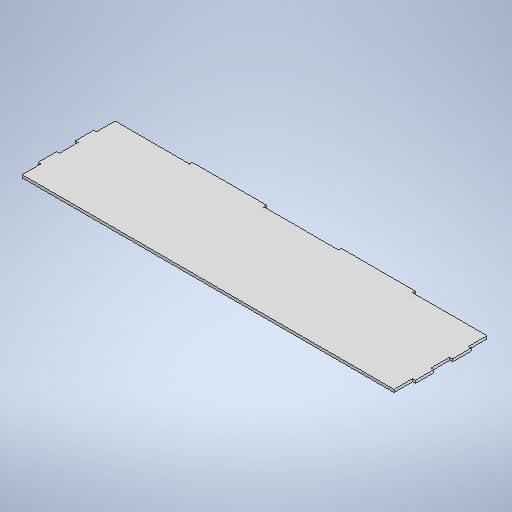
# Autodesk Inventor part: Estante int
Saved by Autodesk Inventor 2025.1 (Build 291241020, 241B)
## iProperties
Created: 2024-11-13
Part Number: Estante int
Material: Generic
Document SubType Name: Modeling
Designer: marco
Density: 1 g/cm^3
Appearance: Default
Author: marco
Autodesk Inventor part; units mm, degrees
ref_plane "YZ Plane" through (0, 0, 0) normal (1, 0, 0) x (0, 1, 0)
ref_plane "XZ Plane" through (0, 0, 0) normal (0, 1, 0) x (-1, 0, 0)
ref_plane "XY Plane" through (0, 0, 0) normal (0, 0, 1) x (1, 0, 0)
sketch "Sketch1" plane through (0, 0, 0) normal (0, 1, 0) x (-1, 0, 0)
  line L0 (0, 0) -> (400, 0)
  line L1 (400, 0) -> (400, -100)
  line L2 (400, -100) -> (0, -100)
  line L3 (320, -103) -> (320, -100)
  line L4 (80, -103) -> (80, -100)
  line L5 (240, -100) -> (240, -103)
  line L6 (160, -103) -> (160, -100)
  line L7 (400, -25) -> (400, -50)
  line L8 (200, 0) -> (200, -100) construction
  line L9 (320, -103) -> (240, -103)
  line L10 (160, -103) -> (80, -103)
  line L11 (400, 0) -> (0, 0)
  line L12 (400, -100) -> (400, 0)
  line L13 (400, -25) -> (400, -50)
  line L14 (400, 0) -> (400, -100)
  line L15 (0, -100) -> (0, 0)
  line L16 (403, -80) -> (400, -80)
  line L17 (403, -80) -> (403, -60)
  line L18 (403, -60) -> (400, -60)
  line L19 (403, -40) -> (400, -40)
  line L20 (403, -40) -> (403, -20)
  line L21 (403, -20) -> (400, -20)
  line L22 (0, -25) -> (0, -50)
  line L23 (0, -25) -> (0, -50)
  line L24 (0, -100) -> (0, 0)
  line L25 (-3, -80) -> (0, -80)
  line L26 (-3, -80) -> (-3, -60)
  line L27 (-3, -60) -> (0, -60)
  line L28 (-3, -40) -> (0, -40)
  line L29 (-3, -40) -> (-3, -20)
  line L30 (-3, -20) -> (0, -20)
  dimension "d1" = 100
  dimension "d7" = 3
  dimension "d8" = 80
  dimension "d17" = 20
  dimension "d18" = 20
  dimension "d19" = 20
  constraints: 62 end point, 13 symmetric about line, 12 point on line, 7 perpendicular, 4 midpoint, 2 equal length, 2 horizontal, 2 vertical
  measures "d1" distance of L0.end L1.end
  measures "d7" distance of L5.start L5.end
  measures "d8" distance of L5.end L6.start
  measures "d17" distance of L16.start L17.end
  measures "d18" distance of L17.end L19.start
  measures "d19" distance of L19.start L20.end
extrude "Extrusion1" add sketch "Sketch1" along normal blind 3
body "Solid1"
